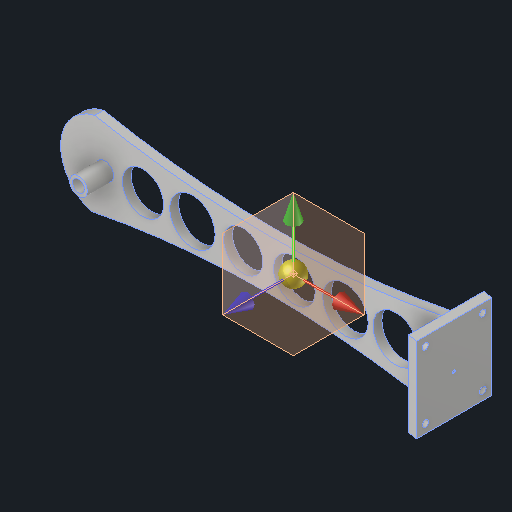
# Autodesk Inventor part: arm
Saved by Autodesk Inventor 2023.4 (Build 274418000, 418)
## iProperties
Created: 2020-06-03
Part Number: arm
Material: Aluminum 6061
Document SubType Name: Modeling
Designer: lenovo
Density: 2.7 g/cm^3
Appearance: Aluminum - Flat
Mass: 46.022 g
Surface Area: 123.884 cm^2
Volume: 17.0452 cm^3
Author: lenovo
Autodesk Inventor part; units mm, degrees
ref_plane "YZ Plane" through (0, 0, 0) normal (1, 0, 0) x (0, 1, 0)
ref_plane "XZ Plane" through (0, 0, 0) normal (0, 1, 0) x (-1, 0, 0)
ref_plane "XY Plane" through (0, 0, 0) normal (0, 0, 1) x (1, 0, 0)
sketch "Sketch1" plane through (0, 0, 0) normal (0, 0, 1) x (1, 0, 0)
  circle A0 centre (-152.5842, 1.6449) radius 20
  circle A1 centre (-2.5848, 1.2498) radius 20
  arc A2 (-157.1373, 21.1198) -> (-0.3077, 21.1198) centre (-78.7225, 413.3584) ccw
  arc A3 (3.2676, -17.8748) -> (-158.9335, -17.3205) centre (-79.1716, -409.2873) ccw
  dimension "d5" = 40
  dimension "d6" = 40
  dimension "d7" = 150
  dimension "d8" = 400
  dimension "d9" = 400
  constraints: 8 point on circle, 4 centre point
  measures "d5" diameter of A0
  measures "d6" diameter of A1
  measures "d7" distance of A1.centre A0.centre
  measures "d8" radius of A2
  measures "d9" radius of A3
extrude "Extrusion1" add sketch "Sketch1" along normal blind 4 contours A2 A0 A3 | A2 A1 A3 A0 | A2 A1 A3
sketch "Sketch2" plane through (0, 0, 4) normal (0, 0, 1) x (1, 0, 0)
  arc A0 (-157.1373, 21.1198) -> (-158.9335, -17.3205) centre (-152.5842, 1.6449) ccw projected
  circle A1 centre (-152.5842, 1.6449) radius 4
  point P0 (0, 0)
  dimension "d12" = 8
  constraints: 1 centre point, 1 coincident
  measures "d12" diameter of A1
extrude "Extrusion2" add sketch "Sketch2" along normal blind 11.9
sketch "Sketch3" plane through (-152.5842, 1.6449, 15.9) normal (0, 0, 1) x (1, 0, 0)
  circle A0 centre (0, 0) radius 2.75
  point P0 (152.5842, -1.6449)
  dimension "d16" = 5.5
  constraints: 1 centre point
  measures "d16" diameter of A0
extrude "Extrusion3" cut sketch "Sketch3" against normal blind 5
sketch "Sketch4" plane through (0, 0, 0) normal (0, 0, -1) x (-1, 0, 0)
  arc A0 (0.3077, 21.1198) -> (-3.2676, -17.8748) centre (2.5848, 1.2498) ccw projected
  line L0 (0.3077, 21.1198) -> (0.3077, -17.1388)
  arc A1 (158.9335, -17.3205) -> (-3.2676, -17.8748) centre (79.1716, -409.2873) ccw projected
  point P0 (0, 0)
  constraints: 2 end point, 1 point on circle, 1 vertical
extrude "Extrusion4" add sketch "Sketch4" along normal blind 15 and the other way blind 19
sketch "Sketch5" plane through (0, 0, -15) normal (0, 0, -1) x (-1, 0, 0)
  arc A0 (0.3077, 21.1198) -> (-3.2676, -17.8748) centre (2.5848, 1.2498) ccw projected
  line L0 (-3.2676, 20.3744) -> (-3.2676, -17.8748)
  point P0 (0, 0)
  constraints: 2 end point, 1 point on circle, 1 vertical
extrude "Extrusion5" cut sketch "Sketch5" against normal blind 35
sketch "Sketch6" plane through (-152.5842, 1.6449, 15.9) normal (0, 0, 1) x (1, 0, 0)
  point P0 (152.5842, -1.6449)
sketch "Sketch7" plane through (-0.3077, -17.1388, 4) normal (-1, 0, 0) x (0, 0, 1)
  point P0 (-4, 17.1388)
sketch "Sketch8" plane through (-0.3077, -17.1388, 4) normal (-1, 0, 0) x (0, 0, 1)
  point P0 (-4, 17.1388)
sketch "Sketch9" plane through (3.2676, -17.8748, -15) normal (1, 0, 0) x (0, 0, -1)
  circle A0 centre (-4, 4) radius 1.475
  circle A1 centre (-4, 34.2492) radius 1.475
  circle A2 centre (-30, 4) radius 1.475
  circle A3 centre (-30, 34.2492) radius 1.475
  line L0 (0, 38.2492) -> (0, 0) projected
  line L1 (-34, 0) -> (-34, 38.2492) projected
  line L2 (0, 0) -> (-34, 0) projected
  line L3 (-34, 38.2492) -> (0, 38.2492) projected
  point P0 (-15, 17.8748)
  dimension "d27" = 2.95
  dimension "d28" = 2.95
  dimension "d29" = 2.95
  dimension "d30" = 2.95
  dimension "d31" = 4
  dimension "d32" = 4
  dimension "d33" = 4
  dimension "d34" = 4
  dimension "d35" = 4
  dimension "d36" = 4
  dimension "d37" = 4
  dimension "d38" = 4
  constraints: 4 centre point
  measures "d27" diameter of A0
  measures "d28" diameter of A1
  measures "d29" diameter of A2
  measures "d30" diameter of A3
  measures "d31" distance from line of L0 A0.centre
  measures "d32" distance from line of L0 A1.centre
  measures "d33" distance from line of L1 A2.centre
  measures "d34" distance from line of L1 A3.centre
  measures "d35" distance from line of L2 A0.centre
  measures "d36" distance from line of L2 A2.centre
  measures "d37" distance from line of L3 A3.centre
  measures "d38" distance from line of L3 A1.centre
extrude "Extrusion6" cut sketch "Sketch9" against normal blind 5 contours A0 | A1 | A2 | A3
sketch "Sketch10" plane through (0, 0, 4) normal (0, 0, 1) x (1, 0, 0)
  point P0 (0, 0)
sketch "Sketch11" plane through (0, 0, 4) normal (0, 0, 1) x (1, 0, 0)
  point P0 (0, 0)
sketch "Sketch12" plane through (0, 0, 4) normal (0, 0, 1) x (1, 0, 0)
  point P0 (0, 0)
sketch "Sketch13" plane through (0, 0, 4) normal (0, 0, 1) x (1, 0, 0)
  circle A0 centre (-113.0156, 1.6449) radius 10.301
  circle A1 centre (-90.0292, 1.6449) radius 8.912
  circle A2 centre (-66.9339, 1.6449) radius 9.4643
  circle A3 centre (-43.8386, 1.6449) radius 10.301
  circle A4 centre (-21.0701, 1.6449) radius 10.301
  circle A5 centre (-135.3483, 1.6449) radius 9.3403
  point P0 (0, 0)
  constraints: 6 centre point
extrude "Extrusion7" cut sketch "Sketch13" against normal blind 10
sketch "Sketch14" plane through (3.2676, -17.8748, -15) normal (1, 0, 0) x (0, 0, -1)
  line L0 (-17.5, 18.3748) -> (-16.5, 18.3748)
  line L1 (-16.5, 18.3748) -> (-16.5, 17.3748)
  line L2 (-16.5, 17.3748) -> (-17.5, 17.3748)
  line L3 (-17.5, 17.3748) -> (-17.5, 18.3748)
  line L4 (-17.5, 18.3748) -> (-16.5, 17.3748) construction
  line L5 (-16.5, 18.3748) -> (-17.5, 17.3748) construction
  point P0 (-15, 17.8748)
  point P1 (-17, 17.8748)
  dimension "d43" = 1
  dimension "d44" = 1
  constraints: 12 end point, 2 midpoint, 2 parallel, 1 horizontal, 1 perpendicular
  measures "d43" distance of L1.end L2.end
  measures "d44" distance of L0.end L1.end
extrude "Extrusion8" cut sketch "Sketch14" against normal blind 0.1
body "Solid1"
